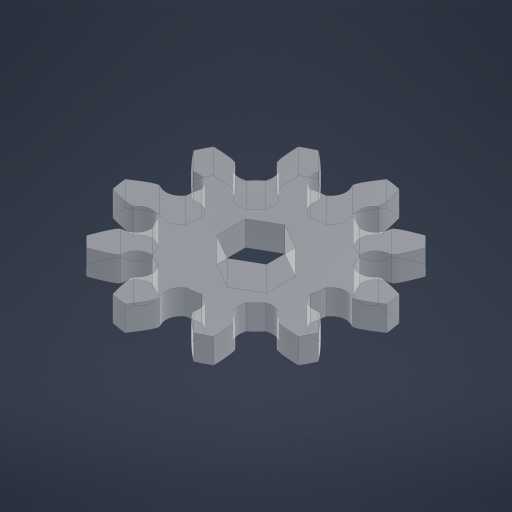
# Autodesk Inventor part: CORL_005_PolyCarbSprocket
Saved by Autodesk Inventor 2024.2 (Build 282272000, 272)
## iProperties
Created: 2024-08-02
Part Number: CORL_005_PolyCarbSprocket
Material: Polycarbonate, Clear
Document SubType Name: Modeling
Designer: Bryan
Density: 1.2 g/cm^3
Appearance: Polycarbonate - Clear
Author: Bryan
Autodesk Inventor part; units mm, degrees
ref_plane "YZ Plane" through (0, 0, 0) normal (1, 0, 0) x (0, 1, 0)
ref_plane "XZ Plane" through (0, 0, 0) normal (0, 1, 0) x (-1, 0, 0)
ref_plane "XY Plane" through (0, 0, 0) normal (0, 0, 1) x (1, 0, 0)
sketch "Sketch1" plane through (0, 0, 0) normal (0, 1, 0) x (-1, 0, 0)
  circle A0 centre (0, 0) radius 25.4 construction
  circle A1 centre (0, 0) radius 19.05
  circle A2 centre (0, 0) radius 30.48
  line L0 (0, 0) -> (25.4, 0) construction
  line L1 (25.4, 0) -> (23.8077, 6.1571) construction
  line L2 (23.8077, 6.1571) -> (0, 0) construction
  arc A3 (24.5906, -0.1364) -> (23.8077, 6.1571) centre (0, 0) ccw construction
  arc A4 (23.8077, 6.1571) -> (18.3771, 16.34) centre (0, 0) ccw construction
  line L3 (18.3771, 16.34) -> (30.3435, 2.8818) construction
  spline S0 degree 2 poles (30.3435, 2.8818) (25.5324, -0.3657) (24.5906, -0.1364) knots 0 0 0 1 1 1
  line L4 (27.7001, 12.7175) -> (6.3501, -29.8112) construction
  line L5 (20.5196, 22.5383) -> (17.5038, -24.9529) construction
  line L6 (24.5906, -0.1364) -> (21.5736, 0.5136) construction
  line L7 (24.5906, -0.1364) -> (19.0117, -1.2073) construction
  line L8 (21.5736, 0.5136) -> (19.0117, -1.2073) construction
  spline S1 degree 2 poles (24.5906, -0.1364) (21.346, 1.699) (19.0117, -1.2073) knots 0 0 0 1 1 1
  line L9 (0, 0) -> (18.8155, -2.9801) construction
  spline S2 degree 2 poles (27.9678, -12.1174) (24.3958, -7.5421) (23.4292, -7.4692) knots 0 0 0 1 1 1
  spline S3 degree 2 poles (23.4292, -7.4692) (19.7763, -8.2121) (18.4543, -4.7267) knots 0 0 0 1 1 1
  spline S4 degree 2 poles (22.8545, 20.1669) (20.8711, 14.7117) (19.9743, 14.3437) knots 0 0 0 1 1 1
  spline S5 degree 2 poles (19.9743, 14.3437) (16.2706, 13.9214) (16.0904, 10.1981) knots 0 0 0 1 1 1
  spline S6 degree 2 poles (29.7489, 6.6358) (24.1697, 8.2378) (23.3449, 7.7286) knots 0 0 0 1 1 1
  spline S7 degree 2 poles (23.3449, 7.7286) (20.8263, 4.9804) (17.7081, 7.0231) knots 0 0 0 1 1 1
  spline S8 degree 2 poles (6.6358, 29.7489) (8.2378, 24.1697) (7.7286, 23.3449) knots 0 0 0 1 1 1
  spline S9 degree 2 poles (7.7286, 23.3449) (4.9804, 20.8263) (7.0231, 17.7081) knots 0 0 0 1 1 1
  spline S10 degree 2 poles (20.1669, 22.8545) (14.7117, 20.8711) (14.3437, 19.9743) knots 0 0 0 1 1 1
  spline S11 degree 2 poles (14.3437, 19.9743) (13.9214, 16.2706) (10.1981, 16.0904) knots 0 0 0 1 1 1
  spline S12 degree 2 poles (-12.1174, 27.9678) (-7.5421, 24.3958) (-7.4692, 23.4292) knots 0 0 0 1 1 1
  spline S13 degree 2 poles (-7.4692, 23.4292) (-8.2121, 19.7763) (-4.7267, 18.4543) knots 0 0 0 1 1 1
  spline S14 degree 2 poles (2.8818, 30.3435) (-0.3657, 25.5324) (-0.1364, 24.5906) knots 0 0 0 1 1 1
  spline S15 degree 2 poles (-0.1364, 24.5906) (1.699, 21.346) (-1.2073, 19.0117) knots 0 0 0 1 1 1
  spline S16 degree 2 poles (-26.2423, 15.504) (-20.4412, 15.3035) (-19.814, 14.5643) knots 0 0 0 1 1 1
  spline S17 degree 2 poles (-19.814, 14.5643) (-18.268, 11.1724) (-14.6712, 12.1515) knots 0 0 0 1 1 1
  spline S18 degree 2 poles (-15.504, 26.2423) (-15.3035, 20.4412) (-14.5643, 19.814) knots 0 0 0 1 1 1
  spline S19 degree 2 poles (-14.5643, 19.814) (-11.1724, 18.268) (-12.1515, 14.6712) knots 0 0 0 1 1 1
  spline S20 degree 2 poles (-30.3435, -2.8818) (-25.5324, 0.3657) (-24.5906, 0.1364) knots 0 0 0 1 1 1
  spline S21 degree 2 poles (-24.5906, 0.1364) (-21.346, -1.699) (-19.0117, 1.2073) knots 0 0 0 1 1 1
  spline S22 degree 2 poles (-27.9678, 12.1174) (-24.3958, 7.5421) (-23.4292, 7.4692) knots 0 0 0 1 1 1
  spline S23 degree 2 poles (-23.4292, 7.4692) (-19.7763, 8.2121) (-18.4543, 4.7267) knots 0 0 0 1 1 1
  spline S24 degree 2 poles (-22.8545, -20.1669) (-20.8711, -14.7117) (-19.9743, -14.3437) knots 0 0 0 1 1 1
  spline S25 degree 2 poles (-19.9743, -14.3437) (-16.2706, -13.9214) (-16.0904, -10.1981) knots 0 0 0 1 1 1
  spline S26 degree 2 poles (-29.7489, -6.6358) (-24.1697, -8.2378) (-23.3449, -7.7286) knots 0 0 0 1 1 1
  spline S27 degree 2 poles (-23.3449, -7.7286) (-20.8263, -4.9804) (-17.7081, -7.0231) knots 0 0 0 1 1 1
  spline S28 degree 2 poles (-6.6358, -29.7489) (-8.2378, -24.1697) (-7.7286, -23.3449) knots 0 0 0 1 1 1
  spline S29 degree 2 poles (-7.7286, -23.3449) (-4.9804, -20.8263) (-7.0231, -17.7081) knots 0 0 0 1 1 1
  spline S30 degree 2 poles (-20.1669, -22.8545) (-14.7117, -20.8711) (-14.3437, -19.9743) knots 0 0 0 1 1 1
  spline S31 degree 2 poles (-14.3437, -19.9743) (-13.9214, -16.2706) (-10.1981, -16.0904) knots 0 0 0 1 1 1
  spline S32 degree 2 poles (12.1174, -27.9678) (7.5421, -24.3958) (7.4692, -23.4292) knots 0 0 0 1 1 1
  spline S33 degree 2 poles (7.4692, -23.4292) (8.2121, -19.7763) (4.7267, -18.4543) knots 0 0 0 1 1 1
  spline S34 degree 2 poles (-2.8818, -30.3435) (0.3657, -25.5324) (0.1364, -24.5906) knots 0 0 0 1 1 1
  spline S35 degree 2 poles (0.1364, -24.5906) (-1.699, -21.346) (1.2073, -19.0117) knots 0 0 0 1 1 1
  spline S36 degree 2 poles (26.2423, -15.504) (20.4412, -15.3035) (19.814, -14.5643) knots 0 0 0 1 1 1
  spline S37 degree 2 poles (19.814, -14.5643) (18.268, -11.1724) (14.6712, -12.1515) knots 0 0 0 1 1 1
  spline S38 degree 2 poles (15.504, -26.2423) (15.3035, -20.4412) (14.5643, -19.814) knots 0 0 0 1 1 1
  spline S39 degree 2 poles (14.5643, -19.814) (11.1724, -18.268) (12.1515, -14.6712) knots 0 0 0 1 1 1
  line L10 (6.35, -3.6662) -> (0, -7.3323)
  line L11 (0, -7.3323) -> (-6.35, -3.6662)
  line L12 (-6.35, -3.6662) -> (-6.35, 3.6662)
  line L13 (-6.35, 3.6662) -> (0, 7.3323)
  line L14 (0, 7.3323) -> (6.35, 3.6662)
  line L15 (6.35, 3.6662) -> (6.35, -3.6662)
  point P0 (24.1568, -7.849)
  point P1 (20.359, -7.1551)
  point P2 (20.549, 14.9297)
  point P3 (17.1515, 13.0961)
  point P4 (24.1568, 7.849)
  point P5 (20.6764, 6.1781)
  point P6 (7.849, 24.1568)
  point P7 (6.1781, 20.6764)
  point P8 (14.9297, 20.549)
  point P9 (13.0961, 17.1515)
  point P10 (-7.849, 24.1568)
  point P11 (-7.1551, 20.359)
  point P12 (0, 25.4)
  point P13 (0.5136, 21.5736)
  point P14 (-20.549, 14.9297)
  point P15 (-17.7553, 12.2651)
  point P16 (-14.9297, 20.549)
  point P17 (-12.2651, 17.7553)
  point P18 (-25.4, 0)
  point P19 (-21.5736, -0.5136)
  point P20 (-24.1568, 7.849)
  point P21 (-20.359, 7.1551)
  point P22 (-20.549, -14.9297)
  point P23 (-17.1515, -13.0961)
  point P24 (-24.1568, -7.849)
  point P25 (-20.6764, -6.1781)
  point P26 (-7.849, -24.1568)
  point P27 (-6.1781, -20.6764)
  point P28 (-14.9297, -20.549)
  point P29 (-13.0961, -17.1515)
  point P30 (7.849, -24.1568)
  point P31 (7.1551, -20.359)
  point P32 (0, -25.4)
  point P33 (-0.5136, -21.5736)
  point P34 (20.549, -14.9297)
  point P35 (17.7553, -12.2651)
  point P36 (14.9297, -20.549)
  point P37 (12.2651, -17.7553)
  point P38 (7.0231, 17.7081)
  point P39 (6.6358, 29.7489)
  point P40 (2.8818, 30.3435)
  point P41 (-1.2073, 19.0117)
  point P42 (-4.7267, 18.4543)
  point P43 (-12.1174, 27.9678)
  point P44 (-15.504, 26.2423)
  point P45 (-12.1515, 14.6712)
  point P46 (-14.6712, 12.1515)
  point P47 (-26.2423, 15.504)
  point P48 (-27.9678, 12.1174)
  point P49 (-18.4543, 4.7267)
  point P50 (-19.0117, 1.2073)
  point P51 (-30.3435, -2.8818)
  point P52 (-29.7489, -6.6358)
  point P53 (-17.7081, -7.0231)
  point P54 (-16.0904, -10.1981)
  point P55 (-22.8545, -20.1669)
  point P56 (-20.1669, -22.8545)
  point P57 (-10.1981, -16.0904)
  point P58 (-7.0231, -17.7081)
  point P59 (-6.6358, -29.7489)
  point P60 (-2.8818, -30.3435)
  point P61 (1.2073, -19.0117)
  point P62 (4.7267, -18.4543)
  point P63 (12.1174, -27.9678)
  point P64 (15.504, -26.2423)
  point P65 (12.1515, -14.6712)
  point P66 (14.6712, -12.1515)
  point P67 (26.2423, -15.504)
  point P68 (27.9678, -12.1174)
  point P69 (18.4543, -4.7267)
  point P70 (19.0117, -1.2073)
  point P71 (29.7489, 6.6358)
  point P72 (17.7081, 7.0231)
  point P73 (16.0904, 10.1981)
  point P74 (22.8545, 20.1669)
  point P75 (20.1669, 22.8545)
  dimension "d0" = 50.8
  dimension "d1" = 38.1
  dimension "d2" = 60.96
  dimension "d3" = 14.5
  dimension "d4" = 18.0088
  dimension "d5" = 6.3597
  dimension "d6" = 6.3597
  dimension "d7" = 11.6491
  dimension "d8" = 75.5
  dimension "d9" = 75.5
  dimension "d10" = 9
  dimension "d13" = 360
  dimension "d15" = 12.7
  constraints: 32 end point, 5 symmetric about line, 4 coincident, 4 point on circle, 2 centre point, 1 equal length, 1 horizontal, 1 horizontal alignment, 1 midpoint, 1 perpendicular, 1 point on line, 1 tangent, 1 vertical, 290 other
  measures "d3" angle of L0 L2
  measures "d4" distance of L3.start L3.end
  measures "d5" distance of L0.end L1.end
  measures "d8" angle of L4 L6
  measures "d9" angle of L5 L7
  measures "d10" angle of L9 L0
  measures "d15" distance between parallel lines of L12 L15
extrude "Extrusion1" add sketch "Sketch1" along normal blind 6.35 contours A1 | A1 S7 S6 A2 S0 S1 | A1 S11 S10 A2 S4 S5 | S3 S2 A2 S36 S37 A1 | A1 S15 S14 A2 S8 S9 | S39 S38 A2 S32 S33 A1 | A1 S19 S18 A2 S12 S13 | S35 S34 A2 S28 S29 A1 | A1 S23 S22 A2 S16 S17 | S31 S30 A2 S24 S25 A1 | A1 S27 S26 A2 S20 S21
equation "\"d0\" = PD"
equation "\"d1\" = RD"
equation "\"d2\" = OD"
equation "\"d3\" = a"
equation "\"d6\" = d5"
equation "\"d7\" = d4 - d5"
equation "\"PD\" = 50.8"
equation "\"a\" = 14.5deg"
equation "\"ded\" = 1.25 * mod"
equation "\"RD\" = PD - 2 * ded"
equation "\"OD\" = PD + 2 * mod"
equation "\"mod\" = 5.08"
body "Solid1"
